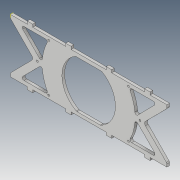
# Autodesk Inventor part: sidePlate
Saved by Autodesk Inventor 2018 (Build 220112000, 112)
## iProperties
Created: 2020-01-09
Part Number: sidePlate
Material: Generic
Document SubType Name: Modeling
Designer: anirudh
Density: 1 g/cm^3
Appearance: Default
Author: anirudh
Autodesk Inventor part; units mm, degrees
ref_plane "YZ Plane" through (0, 0, 0) normal (1, 0, 0) x (0, 1, 0)
ref_plane "XZ Plane" through (0, 0, 0) normal (0, 1, 0) x (-1, 0, 0)
ref_plane "XY Plane" through (0, 0, 0) normal (0, 0, 1) x (1, 0, 0)
sketch "Sketch1" plane through (0, 0, 0) normal (0, 0, 1) x (1, 0, 0)
  line L0 (147.1041, 107.188) -> (114.0841, 107.188)
  line L1 (114.0841, 107.188) -> (114.0841, 112.268)
  line L2 (114.0841, 112.268) -> (103.9229, 112.268)
  line L3 (103.9229, 112.268) -> (103.9229, 107.188)
  line L4 (103.9229, 107.188) -> (41.8453, 107.188)
  line L5 (41.8453, 107.188) -> (41.8453, 112.268)
  line L6 (41.8453, 112.268) -> (31.6853, 112.268)
  line L7 (31.6853, 112.268) -> (31.6853, 107.188)
  line L8 (180.1241, 107.188) -> (180.1241, 112.268)
  line L9 (180.1241, 112.268) -> (190.2841, 112.268)
  line L10 (190.2841, 112.268) -> (190.2841, 107.188)
  line L11 (252.3594, 107.188) -> (252.3594, 112.268)
  line L12 (252.3594, 112.268) -> (262.5194, 112.268)
  line L13 (262.5194, 112.268) -> (262.5194, 107.188)
  line L14 (114.0829, 5.588) -> (114.0829, 0.508)
  line L15 (114.0829, 0.508) -> (103.9229, 0.508)
  line L16 (103.9229, 0.508) -> (103.9229, 5.588)
  line L17 (41.8453, 5.588) -> (41.8453, 0.508)
  line L18 (41.8453, 0.508) -> (31.6853, 0.508)
  line L19 (31.6853, 0.508) -> (31.6853, 5.588)
  line L20 (252.3605, 5.588) -> (252.3605, 0.508)
  line L21 (262.5205, 0.508) -> (262.5205, 5.588)
  line L22 (252.3605, 0.508) -> (262.5205, 0.508)
  line L23 (190.2829, 0.508) -> (190.2829, 5.588)
  line L24 (180.1229, 5.588) -> (180.1229, 0.508)
  line L25 (180.1229, 0.508) -> (190.2829, 0.508)
  line L26 (41.8453, 112.268) -> (31.6853, 112.268)
  line L27 (-0.0012, 107.188) -> (31.6853, 107.188)
  line L28 (41.8453, 107.188) -> (103.9229, 107.188)
  line L29 (114.0841, 112.268) -> (103.9229, 112.268)
  line L30 (262.5194, 112.268) -> (252.3594, 112.268)
  line L31 (190.2841, 112.268) -> (180.1241, 112.268)
  line L32 (114.0841, 107.188) -> (180.1241, 107.188)
  line L33 (190.2841, 107.188) -> (252.3594, 107.188)
  line L34 (262.5194, 107.188) -> (294.207, 107.188)
  line L35 (31.6853, 0.508) -> (41.8453, 0.508)
  line L36 (-0.0012, 5.588) -> (31.6853, 5.588)
  line L37 (103.9229, 0.508) -> (114.0829, 0.508)
  line L38 (41.8453, 5.588) -> (103.9229, 5.588)
  line L39 (180.1229, 0.508) -> (190.2829, 0.508)
  line L40 (252.3605, 0.508) -> (262.5205, 0.508)
  line L41 (114.0829, 5.588) -> (180.1229, 5.588)
  line L42 (190.2829, 5.588) -> (252.3605, 5.588)
  line L43 (262.5205, 5.588) -> (294.207, 5.588)
  line L44 (-0.0012, 107.188) -> (-0.0012, 100.838)
  line L45 (122.6422, 100.33) -> (171.566, 100.33)
  line L46 (-0.0012, 5.588) -> (-0.0012, 11.938)
  arc A0 (169.6444, 11.43) -> (171.566, 100.33) centre (147.1041, 56.388) ccw
  arc A1 (122.6422, 100.33) -> (124.5638, 11.43) centre (147.1041, 56.388) ccw
  line L47 (124.5638, 11.43) -> (169.6444, 11.43)
  arc A2 (40.3794, 52.818) -> (40.3794, 59.958) centre (36.7653, 56.388) ccw
  line L48 (-0.0012, 100.838) -> (40.3794, 59.958)
  line L49 (-0.0012, 11.938) -> (40.3794, 52.818)
  line L50 (-0.0012, 107.188) -> (-0.0012, 100.838)
  line L51 (-0.0012, 11.938) -> (-0.0012, 5.588)
  line L52 (29.2256, 88.8149) -> (17.8511, 100.33)
  line L53 (60.1853, 100.33) -> (60.1853, 57.4722)
  line L54 (60.1853, 57.4722) -> (17.8511, 100.33)
  line L55 (17.8511, 100.33) -> (60.1853, 100.33)
  arc A3 (253.8288, 59.958) -> (253.8288, 52.818) centre (257.4429, 56.388) ccw
  line L56 (294.2094, 100.838) -> (253.8288, 59.958)
  line L57 (294.2094, 11.938) -> (253.8288, 52.818)
  line L58 (264.9826, 88.8149) -> (276.3571, 100.33)
  line L59 (234.0229, 100.33) -> (234.0229, 57.4722)
  line L60 (234.0229, 57.4722) -> (276.3571, 100.33)
  line L61 (276.3571, 100.33) -> (234.0229, 100.33)
  line L62 (-0.0012, 5.588) -> (31.6853, 5.588)
  line L63 (190.2841, 5.588) -> (252.3594, 5.588)
  arc A4 (40.3794, 52.818) -> (40.3794, 59.958) centre (36.7653, 56.388) ccw
  line L64 (29.2256, 23.9611) -> (17.8511, 12.446)
  line L65 (60.1853, 12.446) -> (60.1853, 55.3038)
  line L66 (60.1853, 55.3038) -> (17.8511, 12.446)
  line L67 (17.8511, 12.446) -> (60.1853, 12.446)
  line L68 (234.0229, 12.446) -> (234.0229, 55.3038)
  arc A5 (253.8288, 59.958) -> (253.8288, 52.818) centre (257.4429, 56.388) ccw
  line L69 (234.0229, 55.3038) -> (276.3571, 12.446)
  line L70 (276.3571, 12.446) -> (234.0229, 12.446)
  line L71 (264.9826, 23.9611) -> (276.3571, 12.446)
  line L72 (294.207, 5.588) -> (294.207, 11.9404)
  line L73 (294.207, 100.8356) -> (294.207, 107.188)
  point P0 (0, 0)
  point P1 (262.5194, 5.588)
  dimension "d9" = 6.35
  dimension "d10" = 6.35
  constraints: 148 end point, 51 perpendicular, 16 parallel, 12 point on circle, 6 centre point, 4 horizontal, 2 point on line, 2 vertical, 1 collinear, 1 midpoint
  measures "d9" distance of L27.start L44.end
  measures "d10" distance of L36.start L46.end
extrude "Extrusion1" add sketch "Sketch1" along normal blind 5.08
fillet "Fillet1" radius 3.175 20 edges at (234.0229, 12.446, 2.54) (276.3571, 12.446, 2.54) (234.0229, 55.3038, 2.54) (234.0229, 57.4722, 2.54) (276.3571, 100.33, 2.54) (234.0229, 100.33, 2.54) (17.8511, 12.446, 2.54) (60.1853, 12.446, 2.54) (60.1853, 55.3038, 2.54) (60.1853, 57.4722, 2.54) (60.1853, 100.33, 2.54) (17.8511, 100.33, 2.54) (-0.0012, 100.838, 2.54) (-0.0012, 11.938, 2.54) (122.6422, 100.33, 2.54) (171.566, 100.33, 2.54) (124.5638, 11.43, 2.54) (169.6444, 11.43, 2.54) (294.207, 11.9404, 2.54) (294.207, 100.8356, 2.54)
sketch "Sketch3" plane through (0, 0, 5.08) normal (0, 0, 1) x (1, 0, 0)
  arc A0 (121.8889, 99.9021) -> (123.8608, 11.7894) centre (147.1041, 56.388) ccw projected
  arc A1 (78.0077, 89.3198) -> (78.0077, 23.4562) centre (147.1041, 56.388) ccw projected
  arc A2 (89.3599, 83.619) -> (89.3599, 29.157) centre (147.1041, 56.388) ccw projected
  arc A3 (54.7515, 62.9733) -> (60.1853, 65.2045) centre (57.0103, 65.2045) ccw projected
  arc A4 (71.5944, 100.33) -> (60.1251, 64.589) centre (147.1041, 56.388) ccw
  line L0 (57.0103, 100.33) -> (25.4501, 100.33) projected
  line L1 (49.65, 100.33) -> (71.5944, 100.33)
  line L2 (60.1853, 65.2045) -> (49.65, 100.33)
  arc A5 (234.0229, 65.2045) -> (239.4567, 62.9733) centre (237.1979, 65.2045) ccw
  arc A6 (234.0831, 64.589) -> (222.6138, 100.33) centre (147.1041, 56.388) ccw
  line L3 (244.5582, 100.33) -> (222.6138, 100.33)
  line L4 (234.0229, 65.2045) -> (244.5582, 100.33)
  arc A7 (60.1853, 47.5715) -> (54.7515, 49.8027) centre (57.0103, 47.5715) ccw
  arc A8 (60.1251, 48.187) -> (71.5944, 12.446) centre (147.1041, 56.388) ccw
  line L5 (49.65, 12.446) -> (71.5944, 12.446)
  line L6 (60.1853, 47.5715) -> (49.65, 12.446)
  arc A9 (239.4567, 49.8027) -> (234.0229, 47.5715) centre (237.1979, 47.5715) ccw
  arc A10 (222.6138, 12.446) -> (234.0831, 48.187) centre (147.1041, 56.388) ccw
  line L7 (244.5582, 12.446) -> (222.6138, 12.446)
  line L8 (234.0229, 47.5715) -> (244.5582, 12.446)
  point P0 (0, 0)
  point P1 (237.1979, 100.33)
  point P2 (57.0103, 12.446)
  point P3 (237.1979, 12.446)
  constraints: 22 point on circle, 16 end point, 7 centre point, 1 coincident, 1 collinear, 1 point on line
extrude "Extrusion3" cut sketch "Sketch3" against normal blind 5.08 contours L2 L0 L1 A4 | A6 L3 L4 | A8 L5 L6 | L8 L7 A10
fillet "Fillet3" radius 3.175 8 edges at (71.5944, 100.33, 2.54) (60.1853, 65.2045, 2.54) (71.5944, 12.446, 2.54) (60.1853, 47.5715, 2.54) (222.6138, 12.446, 2.54) (234.0229, 47.5715, 2.54) (222.6138, 100.33, 2.54) (234.0229, 65.2045, 2.54)
ref_plane "Work Plane1" through (-0.0012, 107.188, 0) normal (-1, 0, 0) x (0, 0, 1)
sketch "Sketch5" plane through (0, 0, 5.08) normal (0, 0, 1) x (1, 0, 0)
  arc A0 (40.3794, 52.818) -> (40.3794, 59.958) centre (36.7653, 56.388) ccw projected
  line L0 (31.6853, 107.188) -> (-0.0012, 107.188) projected
  line L1 (-0.0012, 10.6343) -> (-0.0012, 5.588) projected
  line L2 (41.8453, 5.588) -> (103.9229, 5.588) projected
  circle A1 centre (50.5829, 56.388) radius 1.8
  circle A2 centre (72.1094, 101.0412) radius 1.8
  circle A3 centre (72.1094, 11.7348) radius 1.8
  line L3 (180.1241, 107.188) -> (114.0841, 107.188) projected
  arc A4 (170.3474, 11.7894) -> (172.3193, 99.9021) centre (147.1041, 56.388) ccw projected
  circle A5 centre (243.6253, 56.388) radius 1.8
  circle A6 centre (222.0988, 101.0412) radius 1.8
  circle A7 centre (222.0988, 11.7348) radius 1.8
  point P0 (0, 0)
  dimension "d29" = 3.6
  dimension "d30" = 3.6
  constraints: 6 centre point
  measures "d29" diameter of A1
  measures "d30" diameter of A2
extrude "Extrusion5" cut sketch "Sketch5" against normal blind 25.4
body "Solid1"
